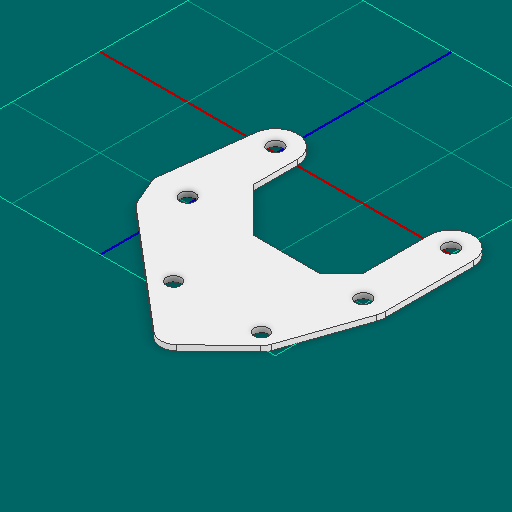
# Autodesk Inventor part: gusset
Saved by Autodesk Inventor 2025 (Build 290162000, 162)
## iProperties
Created: 2024-10-04
Part Number: gusset
Material: Acetal Resin, White
Document SubType Name: Modeling
Designer: Averey Ku
Density: 1.425 g/cm^3
Appearance: Smooth - White
d0: 0.164 in
d1: 0.375 in
d2: 0.500 in
d3: 0.500 in
d4: 0.250 in
d5: 0.250 in
d6: 0.164 in
d7: 0.188 in
d9: 0.125 in
d12: 1.911 in
d14: 0.125 in
d16: 1.000 in
d18: 0.250 in
d17: 1.911 in
Author: Averey Ku
Autodesk Inventor part; units mm, degrees
ref_plane "YZ Plane" through (0, 0, 0) normal (1, 0, 0) x (0, 1, 0)
ref_plane "XZ Plane" through (0, 0, 0) normal (0, 1, 0) x (-1, 0, 0)
ref_plane "XY Plane" through (0, 0, 0) normal (0, 0, 1) x (1, 0, 0)
sketch "main" plane through (0, 0, 0) normal (0, 0, 1) x (1, 0, 0)
  circle A0 centre (9.0037, 34.4943) radius 2.1844
  line L0 (21.7037, 28.1443) -> (9.0037, 15.4443)
  line L1 (34.4037, 28.1443) -> (21.7037, 28.1443)
  circle A1 centre (34.4037, 34.4943) radius 2.1844
  arc A2 (34.4037, 28.1443) -> (34.4037, 40.8443) centre (34.4037, 34.4943) ccw
  arc A3 (-17.5684, -13.257) -> (-15.6972, -14.455) centre (-14.1357, -9.9557) ccw
  circle A4 centre (-14.1357, -9.9557) radius 2.0828
  line L2 (-15.6972, -14.455) -> (6.9217, -22.3047)
  circle A5 centre (-14.1255, 15.4443) radius 2.0828
  line L3 (-29.4913, -0.8595) -> (-17.5684, -13.257)
  arc A6 (-29.6904, 5.5225) -> (-29.4913, -0.8595) centre (-26.0586, 2.4417) ccw
  line L4 (-0.6786, 39.7231) -> (-29.6904, 5.5225)
  line L5 (9.0037, -3.6057) -> (9.0037, 15.4443)
  line L6 (15.3537, -9.9557) -> (34.4037, -9.9557)
  line L7 (15.3537, -9.9557) -> (9.0037, -3.6057)
  circle A7 centre (34.4037, -16.3057) radius 2.1844
  arc A8 (34.4037, -22.6557) -> (34.4037, -9.9557) centre (34.4037, -16.3057) ccw
  circle A9 centre (9.0037, -16.3057) radius 2.1844
  arc A10 (6.9217, -22.3047) -> (9.0037, -22.6557) centre (9.0037, -16.3057) ccw
  line L8 (9.0037, -22.6557) -> (34.4037, -22.6557)
  arc A11 (0.516, 40.5978) -> (-0.6786, 39.7231) centre (1.7426, 37.6693) ccw
  arc A12 (9.1983, 44.0073) -> (8.3903, 43.896) centre (9.0036, 42.4318) ccw
  line L9 (0.516, 40.5978) -> (8.3903, 43.896)
  line L10 (35.1824, 40.7963) -> (9.1983, 44.0073)
  point P0 (6.3419, 6.6617)
  point P1 (9.0037, 28.1443)
  point P2 (0.2724, 40.8443)
  point P3 (-32.4736, 2.2415)
  point P4 (9.0037, -9.9557)
  dimension "d0" = 4.1656
  dimension "d1" = 9.525
  dimension "d2" = 12.7
  dimension "d3" = 12.7
  dimension "d4" = 6.35
  dimension "d5" = 6.35
  dimension "d6" = 4.1656
  dimension "d7" = 4.7625
  dimension "d9" = 3.175
  dimension "d12" = 48.5394
  dimension "d14" = 3.175
  dimension "d16" = 25.4
  dimension "d17" = 48.5291
  dimension "d18" = 6.35
  measures "d0" diameter of A4
  measures "d1" diameter of A3
  measures "d2" distance of L1.end point (9.004, 28.144)
  measures "d3" distance of L5.end point (9.004, 28.144)
  measures "d4" distance of L6.start point (9.004, -9.956)
  measures "d5" distance of L5.start point (9.004, -9.956)
  measures "d6" diameter of A5
  measures "d7" radius of A6
  measures "d9" radius of A11
  measures "d12" horizontal distance of A3.centre A2.centre
  measures "d14" diameter of A12
  measures "d16" distance of A3.centre A5.centre
  measures "d17" horizontal distance of A1.centre A5.centre
  measures "d18" vertical distance of A3.centre A9.centre
sketch "Sketch1" plane through (0, 0, 0) normal (0, 1, 0) x (-1, 0, 0)
  circle A0 centre (0.0003, 25.4) radius 2.1844
  line L0 (-6.3499, 12.7001) -> (-19.0497, 25.4002)
  line L1 (-6.35, 0.0001) -> (-6.3499, 12.7001)
  circle A1 centre (0, 0) radius 2.1844
  arc A2 (-6.35, 0.0001) -> (6.35, -0.0001) centre (0, 0) ccw
  arc A3 (-47.7507, 51.9726) -> (-48.9487, 50.1014) centre (-44.4495, 48.5399) ccw
  circle A4 centre (-44.4495, 48.5399) radius 2.0828
  line L2 (-48.9487, 50.1014) -> (-56.7987, 27.4825)
  circle A5 centre (-19.0495, 48.5293) radius 2.0828
  line L3 (-35.3531, 63.8953) -> (-47.7507, 51.9726)
  arc A6 (-28.9711, 64.0944) -> (-35.3531, 63.8953) centre (-32.0519, 60.4626) ccw
  line L4 (5.2292, 35.0822) -> (-28.9711, 64.0944)
  line L5 (-38.0997, 25.4004) -> (-19.0497, 25.4002)
  line L6 (-44.4498, 19.0505) -> (-44.45, 0.0005)
  line L7 (-44.4498, 19.0505) -> (-38.0997, 25.4004)
  circle A7 centre (-50.8, 0.0005) radius 2.1844
  arc A8 (-57.15, 0.0006) -> (-44.45, 0.0005) centre (-50.8, 0.0005) ccw
  circle A9 centre (-50.7997, 25.4005) radius 2.1844
  arc A10 (-56.7987, 27.4825) -> (-57.1497, 25.4006) centre (-50.7997, 25.4005) ccw
  line L8 (-57.1497, 25.4006) -> (-57.15, 0.0006)
  arc A11 (6.1038, 33.8876) -> (5.2292, 35.0822) centre (3.1753, 32.661) ccw
  arc A12 (9.5133, 25.2052) -> (9.402, 26.0132) centre (7.9378, 25.3999) ccw
  line L9 (6.1038, 33.8876) -> (9.402, 26.0132)
  line L10 (6.3021, -0.7788) -> (9.5133, 25.2052)
  point P0 (0, 0)
  constraints: 1 other
extrude "Extrusion1" add sketch "Sketch1" along normal blind 1.5875
equation "\"d3\" = d2"
equation "\"d5\" = d4"
body "Solid1"
